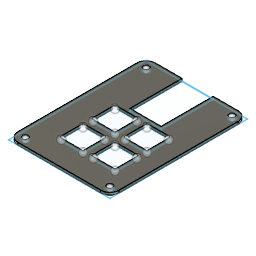
Jackson's ATK Top (Autodesk Fusion 360 design; units mm, degrees)
part number: 2025-12-03-21-45-55-105
part number: 2025-12-03-21-49-20-157
Autodesk Fusion 360 part; units mm, degrees
sketch "Sketch1" plane through (0, 0, 0) normal (0, 0, 1) x (1, 0, 0) in component "Jackson's Editing ATK"
sketch "plate-2025-12-04T02_44_50.134Z" plane through (0, 0, 0) normal (0, 0, 1) x (1, 0, 0)
  line L0 (3.025, -2.525) -> (16.025, -2.525)
  line L1 (3.025, -16.525) -> (16.025, -16.525)
  line L2 (2.525, -3.025) -> (2.525, -16.025)
  line L3 (16.525, -3.025) -> (16.525, -16.025)
  arc A0 (3.025, -2.525) -> (2.525, -3.025) centre (3.025, -3.025) ccw
  arc A1 (16.525, -3.025) -> (16.025, -2.525) centre (16.025, -3.025) ccw
  arc A2 (2.525, -16.025) -> (3.025, -16.525) centre (3.025, -16.025) ccw
  arc A3 (16.025, -16.525) -> (16.525, -16.025) centre (16.025, -16.025) ccw
  line L4 (22.075, -2.525) -> (35.075, -2.525)
  line L5 (22.075, -16.525) -> (35.075, -16.525)
  line L6 (21.575, -3.025) -> (21.575, -16.025)
  line L7 (35.575, -3.025) -> (35.575, -16.025)
  arc A4 (22.075, -2.525) -> (21.575, -3.025) centre (22.075, -3.025) ccw
  arc A5 (35.575, -3.025) -> (35.075, -2.525) centre (35.075, -3.025) ccw
  arc A6 (21.575, -16.025) -> (22.075, -16.525) centre (22.075, -16.025) ccw
  arc A7 (35.075, -16.525) -> (35.575, -16.025) centre (35.075, -16.025) ccw
  line L8 (3.025, -21.575) -> (16.025, -21.575)
  line L9 (3.025, -35.575) -> (16.025, -35.575)
  line L10 (2.525, -22.075) -> (2.525, -35.075)
  line L11 (16.525, -22.075) -> (16.525, -35.075)
  arc A8 (3.025, -21.575) -> (2.525, -22.075) centre (3.025, -22.075) ccw
  arc A9 (16.525, -22.075) -> (16.025, -21.575) centre (16.025, -22.075) ccw
  arc A10 (2.525, -35.075) -> (3.025, -35.575) centre (3.025, -35.075) ccw
  arc A11 (16.025, -35.575) -> (16.525, -35.075) centre (16.025, -35.075) ccw
  line L12 (22.075, -21.575) -> (35.075, -21.575)
  line L13 (22.075, -35.575) -> (35.075, -35.575)
  line L14 (21.575, -22.075) -> (21.575, -35.075)
  line L15 (35.575, -22.075) -> (35.575, -35.075)
  arc A12 (22.075, -21.575) -> (21.575, -22.075) centre (22.075, -22.075) ccw
  arc A13 (35.575, -22.075) -> (35.075, -21.575) centre (35.075, -22.075) ccw
  arc A14 (21.575, -35.075) -> (22.075, -35.575) centre (22.075, -35.075) ccw
  arc A15 (35.075, -35.575) -> (35.575, -35.075) centre (35.075, -35.075) ccw
sketch "Sketch2" plane through (0, 0, 0) normal (0, 0, 1) x (1, 0, 0)
  line L0 (-12.675, 31.185) -> (47.695, 31.185)
  line L1 (47.695, 31.185) -> (47.695, -50.775)
  line L2 (47.695, -50.775) -> (-12.675, -50.775)
  line L3 (-12.675, -50.775) -> (-12.675, 31.185)
  line L4 (8.773, 31.185) -> (27.273, 31.185)
  line L5 (27.273, 31.185) -> (27.273, 0.185)
  line L6 (27.273, 0.185) -> (8.773, 0.185)
  line L7 (8.773, 0.185) -> (8.773, 31.185)
  circle A0 centre (42.695, 27) radius 1.7
  circle A1 centre (-7.675, 26.185) radius 1.7
  circle A2 centre (-7.675, -45.775) radius 1.7
  circle A3 centre (42.695, -45.775) radius 1.7
  dimension "d12" = 60.37
  dimension "d13" = 81.96
  dimension "d16" = 21.448
  dimension "d17" = 18.5
  dimension "d18" = 31
  dimension "d19" = 3.4
  dimension "d20" = 5
  dimension "d21" = 3.4
  dimension "d22" = 5
  dimension "d23" = 5
  dimension "d24" = 3.4
  dimension "d25" = 5
  dimension "d26" = 5
  dimension "d27" = 3.4
  dimension "d28" = 5
  dimension "d29" = 5
  constraint horizontal L0
  constraint vertical L1
  constraint horizontal L2
  constraint vertical L3
  constraint horizontal L4
  constraint vertical L5
  constraint horizontal L6
  constraint vertical L7
  constraint coincident L0 L4.start
  measures "d12" distance of L1 L3
  measures "d13" distance of L0 L2
  measures "d16" distance of L3 L7
  measures "d17" distance of L5 L7
  measures "d18" distance of L0 L6
  measures "d19" diameter of A0
  measures "d20" distance of L1 A0.centre
  measures "d21" diameter of A1
  measures "d22" distance of L3 A1.centre
  measures "d23" distance of L0 A1.centre
  measures "d24" diameter of A2
  measures "d25" distance of L3 A2.centre
  measures "d26" distance of L2 A2.centre
  measures "d27" diameter of A3
  measures "d28" distance of L2 A3.centre
  measures "d29" distance of L1 A3.centre
extrude "Extrude1" add sketch "Sketch2" along normal blind 1.5 contours L0 L1 L2 L3 L5 L6 L7 makes body 1
extrude "Extrude2" add sketch "Sketch2" along normal blind 1.5 separate body contours L0 L1 L2 L3 L5 L6 L7 makes body 2
combine "Combine1" operation add target body 1 tool bodies 2
extrude "Extrude3" cut sketch "plate-2025-12-04T02_44_50.134Z" along normal blind 1.5 bodies 1
fillet "Fillet1" radius 5.5 1 edges at (47.695, -50.775, 0.75) on bodies 1
fillet "Fillet2" radius 5.5 1 edges at (47.695, 31.185, 0.75) on bodies 1
fillet "Fillet3" radius 5.5 1 edges at (-12.675, -50.775, 0.75) on bodies 1
fillet "Fillet4" radius 5.5 1 edges at (-12.675, 31.185, 0.75) on bodies 1
sketch "Sketch3" plane through (0, 0, 0) normal (0, 0, 1) x (1, 0, 0)
  line L0 (37.8851, -35.3799) -> (0.8851, -35.3799) construction
  line L1 (0.8851, -35.3799) -> (0.8851, -49.3799) construction
  line L2 (0.8851, -49.3799) -> (37.8851, -49.3799) construction
  line L3 (37.8851, -49.3799) -> (37.8851, -35.3799) construction
  dimension "d44" = 3
  text T0 "Jacksons \nEditing\nATK V1" font "Arial" height 3 align left top in box 37 x 14 at (37.8851, -35.3799) x (-1, 0) y (0, -1) spacing 1 kerned
extrude "Extrude4" cut sketch "Sketch3" along normal blind 0.2 text T0 bodies 1
component "Jackson's Editing ATK" placed x (1, 0, 0) y (0, 1, 0) z (0, 0, 1) at (0, 0, 0)
equation "d45 = 'Jacksons  Editing ATK V1'"
